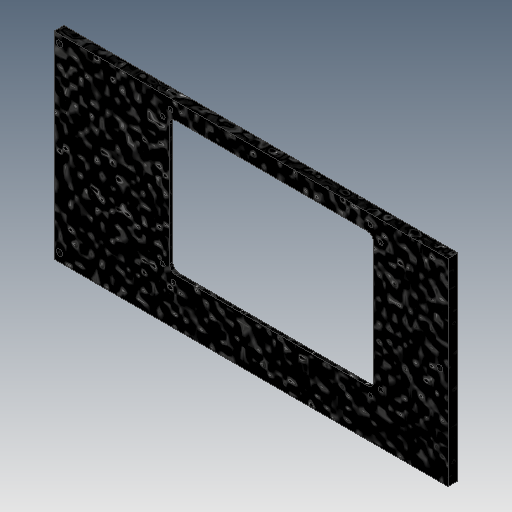
# Autodesk Inventor part: 04_OPENTRONS_Microscope_wellplate_base
Saved by Autodesk Inventor 2019.4 (Build 234330000, 330)
## iProperties
Created: 2020-11-05
Part Number: 04_OPENTRONS_Microscope_wellplate_base
Material: Generic
Document SubType Name: Modeling
Designer: diederichbenedict
Density: 1 g/cm^3
Appearance: Black
Author: diederichbenedict
Autodesk Inventor part; units mm, degrees
ref_plane "YZ Plane" through (0, 0, 0) normal (1, 0, 0) x (0, 1, 0)
ref_plane "XZ Plane" through (0, 0, 0) normal (0, 1, 0) x (-1, 0, 0)
ref_plane "XY Plane" through (0, 0, 0) normal (0, 0, 1) x (1, 0, 0)
sketch "Sketch1" plane through (0, 0, 0) normal (0, 0, 1) x (1, 0, 0)
  line L0 (-127.4, 49.6) -> (111.9, 49.6)
  line L1 (111.9, 49.6) -> (111.9, -70.3)
  line L2 (111.9, -70.3) -> (-127.4, -70.3)
  line L3 (-127.4, -70.3) -> (-127.4, 49.6)
  line L4 (-154.2, -74.9) -> (-154.2, -103.9) construction
  line L5 (64.8, 41.6) -> (16.1, 41.6) construction
  arc A0 (68.7, 37.7) -> (64.8, 41.6) centre (64.8, 37.7) ccw construction
  line L6 (68.7, -39.9) -> (68.7, 37.7) construction
  arc A1 (64.8, -43.8) -> (68.7, -39.9) centre (64.8, -39.9) ccw construction
  line L7 (16.1, -43.8) -> (64.8, -43.8) construction
  line L8 (16.1, -42.3) -> (16.1, -43.8) construction
  line L9 (60.6858, -42.3) -> (16.1, -42.3) construction
  arc A2 (60.6858, -42.3) -> (61.4636, -41.9778) centre (60.6858, -41.2) ccw construction
  line L10 (66.8778, -36.5636) -> (61.4636, -41.9778) construction
  arc A3 (66.8778, -36.5636) -> (67.2, -35.7858) centre (66.1, -35.7858) ccw construction
  line L11 (67.2, 33.5858) -> (67.2, -35.7858) construction
  arc A4 (67.2, 33.5858) -> (66.8778, 34.3636) centre (66.1, 33.5858) ccw construction
  line L12 (61.4636, 39.7778) -> (66.8778, 34.3636) construction
  arc A5 (61.4636, 39.7778) -> (60.6858, 40.1) centre (60.6858, 39) ccw construction
  line L13 (16.1, 40.1) -> (60.6858, 40.1) construction
  line L14 (16.1, 41.6) -> (16.1, 40.1) construction
  line L15 (-6.3, 41.6) -> (-55, 41.6) construction
  line L16 (-6.3, 40.1) -> (-6.3, 41.6) construction
  line L17 (-55.3, 40.1) -> (-6.3, 40.1) construction
  arc A6 (-55.3, 40.1) -> (-57.4, 38) centre (-55.3, 38) ccw construction
  line L18 (-57.4, -40.2) -> (-57.4, 38) construction
  arc A7 (-57.4, -40.2) -> (-55.3, -42.3) centre (-55.3, -40.2) ccw construction
  line L19 (-6.3, -42.3) -> (-55.3, -42.3) construction
  line L20 (-6.3, -43.8) -> (-6.3, -42.3) construction
  line L21 (-55, -43.8) -> (-6.3, -43.8) construction
  arc A8 (-58.9, -39.9) -> (-55, -43.8) centre (-55, -39.9) ccw construction
  line L22 (-58.9, 37.7) -> (-58.9, -39.9) construction
  arc A9 (-55, 41.6) -> (-58.9, 37.7) centre (-55, 37.7) ccw construction
  line L23 (62.7, -41.8) -> (-53.4, -41.8)
  line L24 (-57.4, -37.8) -> (-57.4, 35.6)
  line L25 (-53.4, 39.6) -> (62.7, 39.6)
  line L26 (66.7, 35.6) -> (66.7, -37.8)
  arc A10 (-53.4, 39.6) -> (-57.4, 35.6) centre (-53.4, 35.6) ccw
  arc A11 (-57.4, -37.8) -> (-53.4, -41.8) centre (-53.4, -37.8) ccw
  arc A12 (66.7, 35.6) -> (62.7, 39.6) centre (62.7, 35.6) ccw
  arc A13 (62.7, -41.8) -> (66.7, -37.8) centre (62.7, -37.8) ccw
  line L27 (111.9, -36.0431) -> (111.9, -26.0431) projected
  dimension "d54" = 4
  dimension "d55" = 2
  dimension "d56" = 2
  dimension "d67" = 10
  dimension "d68" = 28
  dimension "d70" = 70
  dimension "d72" = 0
  constraints: 16 end point, 8 point on circle, 8 tangent, 4 centre point, 4 parallel, 3 equal radius, 2 horizontal, 2 perpendicular
  measures "d54" radius of A10
  measures "d55" distance between parallel lines of L25 L15
  measures "d56" distance between parallel lines of L26 L6
  measures "d67" distance between parallel lines of L0 L25
  measures "d68" distance between parallel lines of L2 L9
  measures "d70" distance between parallel lines of L3 L24
  measures "d72" distance between parallel lines of L27 L1
extrude "Extrusion1" add sketch "Sketch1" along normal blind 2
hole "Hole1" at (71, 37.7, 0) at (64.8, 43.9, 0) at (71, -39.9, 0) at (64.8, -46.1, 0) at (-55, -46.3, 0) at (-61.4, -39.9, 0) at (-61.4, 37.7, 0) at (-56.5875, 43.9, 0) direction (0, 0, 1) diameter 2.9 end through all
sketch "Sketch10" plane through (0, 0, 0) normal (0, 0, -1) x (-1, 0, 0)
  circle A0 centre (61.4, 37.7) radius 1.45 projected
  circle A1 centre (55, -46.3) radius 1.45 projected
  circle A2 centre (-71, -39.9) radius 1.45 projected
  circle A3 centre (-71, 37.7) radius 1.45 projected
  circle A4 centre (-64.8, 43.9) radius 1.45 projected
  circle A5 centre (-64.8, -46.1) radius 1.45 projected
  circle A6 centre (61.4, -39.9) radius 1.45 projected
  circle A7 centre (56.5875, 43.9) radius 1.45 projected
  arc A8 (57.4, 35.6) -> (53.4, 39.6) centre (53.4, 35.6) ccw projected
  line L0 (57.4, 35.6) -> (57.4, -37.8) projected
  arc A9 (53.4, -41.8) -> (57.4, -37.8) centre (53.4, -37.8) ccw projected
  line L1 (53.4, -41.8) -> (-62.7, -41.8) projected
  arc A10 (-66.7, -37.8) -> (-62.7, -41.8) centre (-62.7, -37.8) ccw projected
  line L2 (-66.7, -37.8) -> (-66.7, 35.6) projected
  arc A11 (-62.7, 39.6) -> (-66.7, 35.6) centre (-62.7, 35.6) ccw projected
  line L3 (-62.7, 39.6) -> (53.4, 39.6) projected
  line L4 (127.4, 49.6) -> (-111.9, 49.6) projected
  line L5 (-111.9, 49.6) -> (-111.9, -70.3) projected
  line L6 (-111.9, -70.3) -> (127.4, -70.3) projected
  line L7 (127.4, -70.3) -> (127.4, 49.6) projected
  line L8 (-104.9, -63.3) -> (-104.9, 42.6)
  line L9 (-104.9, 42.6) -> (120.4, 42.6)
  line L10 (120.4, 42.6) -> (120.4, -63.3)
  line L11 (120.4, -63.3) -> (-104.9, -63.3)
  point P0 (0, 0)
  dimension "d73" = 7
  constraints: 8 end point, 3 other
  measures "d73" distance between parallel lines of L5 L8
extrude "Extrusion7" add sketch "Sketch10" along normal blind 4 contours L7 L6 L5 L4
sketch "Sketch11" plane through (0, 0, -4) normal (0, 0, -1) x (-1, 0, 0)
  circle A0 centre (-106.9, -10.4) radius 1.9 projected
  circle A1 centre (124.1, 44.6) radius 1.9 projected
  circle A2 centre (124.1, -65.2236) radius 1.9 projected
  point P0 (0, 0)
extrude "Extrusion8" cut sketch "Sketch11" against normal through all
body "Solid1"
